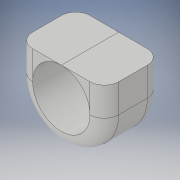
# Autodesk Inventor part: trzym
Saved by Autodesk Inventor 2019 (Build 230136000, 136)
## iProperties
Created: 2020-01-12
Part Number: trzym
Material: Ogólny
Document SubType Name: Modeling
Designer: Karolina
Density: 1 g/cm^3
Appearance: Domyślna
Author: Karolina
Autodesk Inventor part; units mm, degrees
ref_plane "YZ Plane" through (0, 0, 0) normal (1, 0, 0) x (0, 1, 0)
ref_plane "XZ Plane" through (0, 0, 0) normal (0, 1, 0) x (-1, 0, 0)
ref_plane "XY Plane" through (0, 0, 0) normal (0, 0, 1) x (1, 0, 0)
sketch "Szkic1" plane through (0, 0, 0) normal (0, 0, 1) x (1, 0, 0)
  line L0 (0, -1) -> (0, 0.75) construction
  line L1 (-1.05, 0) -> (1.05, 0) construction
  circle A0 centre (0, 0) radius 0.5
  line L2 (0.75, -0.5) -> (-0.75, -0.5) construction
  line L3 (-0.75, -0.5) -> (-0.75, 0.5) construction
  line L4 (-0.75, 0.5) -> (0.75, 0.5)
  line L5 (0.75, 0.5) -> (0.75, -0.5) construction
  line L6 (0.75, -0.5) -> (-0.75, 0.5) construction
  line L7 (-0.75, -0.5) -> (0.75, 0.5) construction
  line L8 (-0.75, 0) -> (-0.75, 0.5)
  line L9 (0.75, 0.5) -> (0.75, 0)
  arc A1 (-0.75, 0) -> (0.75, 0) centre (0, 0) ccw
  point P0 (0, 0)
  dimension "d5" = 1
  dimension "d7" = 1.5
  constraints: 16 end point, 5 midpoint, 3 tangent, 2 centre point, 2 coincident, 2 parallel, 2 perpendicular, 2 point on circle, 1 horizontal
  measures "d5" diameter of A0
  measures "d7" distance between parallel lines of L5 L3
extrude "Wyciągnięcie proste1" add sketch "Szkic1" along normal blind 1
fillet "Zaokrąglenie1" radius 0.25 6 edges at (-0.75, 0.25, 0) (0.75, 0.25, 0) (0, -0.75, 0) (0.75, 0.25, 1) (-0.75, 0.25, 1) (0, -0.75, 1)
